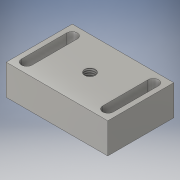
# Autodesk Inventor part: Track Foot
Saved by Autodesk Inventor 2016 (Build 200138000, 138)
## iProperties
Created: 2015-06-03
Part Number: Track Foot
Material: Aluminum 6061
Document SubType Name: Modeling
Designer: Dennis
Density: 2.7 g/cm^3
Appearance: Aluminum - Polished
Mass: 106.159 g
Surface Area: 108.464 cm^2
Volume: 39.318 cm^3
Author: Dennis
Autodesk Inventor part; units mm, degrees
ref_plane "YZ Plane" through (0, 0, 0) normal (1, 0, 0) x (0, 1, 0)
ref_plane "XZ Plane" through (0, 0, 0) normal (0, 1, 0) x (-1, 0, 0)
ref_plane "XY Plane" through (0, 0, 0) normal (0, 0, 1) x (1, 0, 0)
sketch "Sketch1" plane through (0, 0, 0) normal (0, 0, 1) x (1, 0, 0)
  line L0 (0, 0) -> (63.5, 0)
  line L1 (63.5, 0) -> (63.5, 19.05)
  line L2 (63.5, 19.05) -> (0, 19.05)
  line L3 (0, 19.05) -> (0, 0)
  dimension "d2" = 63.5
  dimension "d3" = 19.05
  constraints: 8 end point, 2 parallel, 1 horizontal, 1 perpendicular
  measures "d2" distance of L0.start L0.end
  measures "d3" distance of L0.end L1.end
extrude "Stock Block" add sketch "Sketch1" along normal blind 41.275
sketch "Sketch2" plane through (0, 19.05, 0) normal (0, 1, 0) x (1, 0, 0)
  line L0 (63.5, 0) -> (0, 0) projected
  line L1 (0, 0) -> (0, -41.275) projected
  point P0 (31.75, -20.6375)
  dimension "d4" = 20.6375
  dimension "d5" = 31.75
  measures "d4" distance from line of point (31.75, -20.638) L0
  measures "d5" distance from line of point (31.75, -20.638) L1
hole "Mounting Hole" at (31.75, 19.05, 20.6375) direction (0, -1, 0) diameter 6.6548 end through all
sketch "Sketch3" plane through (0, 19.05, 0) normal (0, 1, 0) x (1, 0, 0)
  line L0 (6.35, -34.798) -> (6.35, -6.477) construction
  line L1 (3.048, -34.798) -> (3.048, -6.477)
  line L2 (9.652, -6.477) -> (9.652, -34.798)
  arc A0 (3.048, -34.798) -> (9.652, -34.798) centre (6.35, -34.798) ccw
  arc A1 (9.652, -6.477) -> (3.048, -6.477) centre (6.35, -6.477) ccw
  line L3 (0, 0) -> (0, -41.275) projected
  line L4 (63.5, -41.275) -> (0, -41.275) projected
  line L5 (63.5, 0) -> (0, 0) projected
  circle A2 centre (31.75, -20.6375) radius 3.3274 projected
  line L6 (31.75, -20.6375) -> (31.75, 0) construction
  line L7 (57.15, -34.798) -> (57.15, -6.477) construction
  line L8 (60.452, -34.798) -> (60.452, -6.477)
  line L9 (53.848, -6.477) -> (53.848, -34.798)
  arc A3 (53.848, -34.798) -> (60.452, -34.798) centre (57.15, -34.798) ccw
  arc A4 (60.452, -6.477) -> (53.848, -6.477) centre (57.15, -6.477) ccw
  point P0 (6.35, -20.6375)
  point P1 (57.15, -20.6375)
  dimension "d13" = 6.604
  dimension "d15" = 3.175
  dimension "d16" = 3.175
  dimension "d24" = 25.4
  constraints: 18 end point, 8 point on circle, 7 symmetric about line, 4 centre point, 4 tangent, 2 midpoint, 1 parallel, 1 vertical, 2 other
  measures "d13" distance between parallel lines of L1 L2
  measures "d15" distance edge to line of A0 L4
  measures "d16" distance edge to line of A1 L5
  measures "d24" distance of L6.start point (6.35, -20.638)
extrude "Slots" cut sketch "Sketch3" against normal up to surface (19.05 mm away) contours L1 A1 L2 A0 | A3 L9 A4 L8
body "Solid1"
